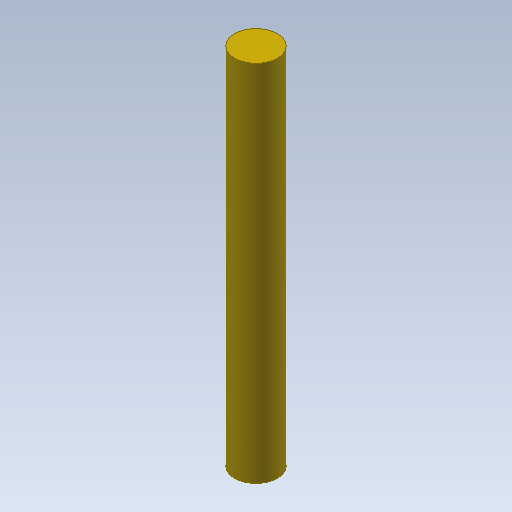
# Autodesk Inventor part: Locking Pin Lever
Saved by Autodesk Inventor 2020 (Build 240168000, 168)
## iProperties
Created: 2012-11-06
Part Number: Locking Pin Lever
Document SubType Name: Modeling
Designer: Lance
Density: 1 g/cm^3
Material: Generic
Appearance: Glossy - Gold
Mass: 0.0534071 g
Surface Area: 1.13097 cm^2
Volume: 0.0534071 cm^3
Author: Lance
Autodesk Inventor part; units mm, degrees
ref_plane "YZ Plane" through (0, 0, 0) normal (1, 0, 0) x (0, 1, 0)
ref_plane "XZ Plane" through (0, 0, 0) normal (0, 1, 0) x (-1, 0, 0)
ref_plane "XY Plane" through (0, 0, 0) normal (0, 0, 1) x (1, 0, 0)
sketch "Sketch1" plane through (0, 0, 0) normal (0, 0, 1) x (1, 0, 0)
  line L0 (0, 8.5) -> (0, -8.5)
  line L1 (0, -8.5) -> (1, -8.5)
  line L2 (1, -8.5) -> (1, 8.5)
  line L3 (1, 8.5) -> (0, 8.5)
  point P0 (0, 0)
  point P1 (0, 0)
  dimension "d1" = 2
  dimension "d5" = 17
  constraints: 8 end point, 2 perpendicular, 1 coincident, 1 midpoint, 1 parallel, 1 vertical
  measures "d1" diameter of L2 L0
  measures "d5" distance between parallel lines of L1 L3
revolve "Revolution1" add sketch "Sketch1" angle 360 about axis through (0, 8.5, 0) along (0, -1, 0)
body "Solid1"
